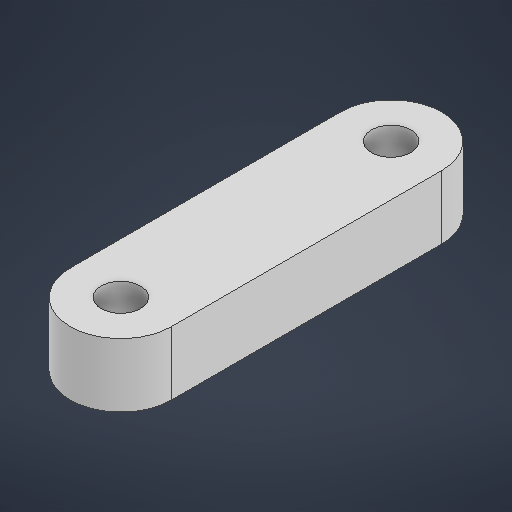
# Autodesk Inventor part: FourBarSection
Saved by Autodesk Inventor 2025 (Build 290162000, 162)
## iProperties
Created: 2024-05-20
Part Number: FourBarSection
Material: Generic
Document SubType Name: Modeling
Designer: avsar
Density: 1 g/cm^3
Appearance: Default
Author: avsar
Autodesk Inventor part; units mm, degrees
ref_plane "YZ Plane" through (0, 0, 0) normal (1, 0, 0) x (0, 1, 0)
ref_plane "XZ Plane" through (0, 0, 0) normal (0, 1, 0) x (-1, 0, 0)
ref_plane "XY Plane" through (0, 0, 0) normal (0, 0, 1) x (1, 0, 0)
sketch "Sketch1" plane through (0, 0, 0) normal (0, 1, 0) x (-1, 0, 0)
  line L0 (9, 33) -> (-9, 33)
  line L1 (-9, 33) -> (-9, -33)
  line L2 (-9, -33) -> (9, -33)
  line L3 (9, -33) -> (9, 33)
  line L4 (9, 33) -> (-9, -33) construction
  line L5 (-9, 33) -> (9, -33) construction
  circle A0 centre (0, -24) radius 3.5
  line L6 (9, 0) -> (-9, 0) construction
  circle A1 centre (0, 24) radius 3.5
  point P0 (0, 0)
  dimension "d0" = 18
  dimension "d1" = 66
  dimension "d3" = 7
  dimension "d4" = 24
  constraints: 14 end point, 4 midpoint, 2 centre point, 2 parallel, 1 horizontal, 1 perpendicular, 1 symmetric about line, 1 vertical alignment, 1 other
  measures "d0" distance of L2.end L1.end
  measures "d1" distance of L0.end L1.end
  measures "d3" diameter of A0
  measures "d4" distance of A0.centre point (0, 0)
extrude "Extrusion1" add sketch "Sketch1" along normal blind 11.3
fillet "Fillet1" radius 9 4 edges at (-9, 5.65, 33) (9, 5.65, 33) (9, 5.65, -33) (-9, 5.65, -33)
body "Solid1"
